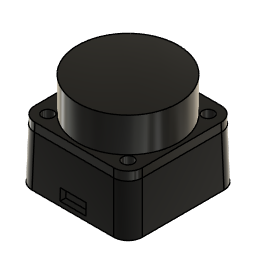
OKDO Lidar v2 (Autodesk Fusion 360 design; units mm, degrees)
Autodesk Fusion 360 part; units mm, degrees
note: some values were not read from the file. Set by a fixed rule: which face or edge a step refers to.
sketch "Sketch1" plane through (0, 0, 0) normal (0, 0, 1) x (1, 0, 0)
  line L0 (18.75, -18.75) -> (-18.75, -18.75)
  line L1 (-18.75, -18.75) -> (-18.75, 18.75)
  line L2 (-18.75, 18.75) -> (18.75, 18.75)
  line L3 (18.75, 18.75) -> (18.75, -18.75)
  line L4 (18.75, -18.75) -> (-18.75, 18.75) construction
  line L5 (-18.75, -18.75) -> (18.75, 18.75) construction
  dimension "d1" = 37.5
  dimension "d2" = 37.5
  constraint horizontal L0
  constraint perpendicular L0 L1
  constraint parallel L0 L2
  constraint parallel L1 L3
  constraint coincident L4 origin
  constraint coincident L5 origin
  measures "d1" distance of L1.end L2.end
  measures "d2" distance of L0.end L1.end
extrude "Extrude1" add sketch "Sketch1" against normal blind 20.5 makes body 1
sketch "Sketch2" plane through (0, 0, -20.5) normal (0, 0, -1) x (1, 0, 0)
  line L0 (-18.75, -18.75) -> (18.75, -18.75)
  line L1 (18.75, -18.75) -> (18.75, 18.75)
  line L2 (18.75, 18.75) -> (-18.75, 18.75)
  line L3 (-18.75, 18.75) -> (-18.75, -18.75)
  line L4 (19.25, 19.25) -> (-19.25, 19.25)
  line L5 (-19.25, 19.25) -> (-19.25, -19.25)
  line L6 (-19.25, -19.25) -> (19.25, -19.25)
  line L7 (19.25, -19.25) -> (19.25, 19.25)
  line L8 (19.25, 19.25) -> (-19.25, -19.25) construction
  line L9 (-19.25, 19.25) -> (19.25, -19.25) construction
  dimension "d5" = 38.5
  dimension "d6" = 38.5
  constraint horizontal L4
  constraint perpendicular L4 L5
  constraint parallel L4 L6
  constraint parallel L5 L7
  constraint coincident L8 origin
  constraint coincident L9 origin
  measures "d5" distance of L5.end L6.end
  measures "d6" distance of L4.end L5.end
sketch "Sketch3" plane through (0, -18.75, 0) normal (0, -1, 0) x (1, 0, 0)
  line L0 (18.75, 0) -> (-18.75, 0)
  line L1 (-18.75, 0) -> (-18.75, -20.5)
  line L2 (-18.75, -20.5) -> (18.75, -20.5)
  line L3 (18.75, -20.5) -> (18.75, 0)
  line L4 (-18.75, 0) -> (-19.25, -20.5)
  line L5 (-19.25, -20.5) -> (-18.75, -20.5)
  constraint coincident L0.end L1.start
  constraint coincident L1.end L2.start
extrude "Extrude2" add sketch "Sketch3" against normal blind 37.5 contours L1 L4 L5 bodies 1
pattern_circular "C-Pattern1" count 4 over 360 about axis through (0, 0, 1.75) along (0, 0, 1) of bodies 1 makes body 2 at (-6.25, -18.9167, -6.8333) makes body 3 at (18.9167, -6.25, -6.8333) makes body 4 at (6.25, 18.9167, -6.8333)
combine "Combine1" operation add target body 1 tool bodies 2 3 4
extrude "Extrude3" add 1 faces at (18.75, -18.9167, -13.6667) along direction (1, 0, 0) blind 0.9 on bodies 1 bodies 1
extrude "Extrude4" cut 1 faces at (19.2167, -18.75, -6.8333) along direction (0, -1, 0) blind 1.5 on bodies 1 bodies 1
extrude "Extrude5" add 1 faces at (18.75, 18.9167, -13.6667) along direction (1, 0, 0) blind 1 on bodies 1 bodies 1
extrude "Extrude6" add 2 faces at (-18.75, 18.9167, -13.6667) (-18.75, -18.9167, -13.6667) along direction (-1, 0, 0) blind 2.5 on bodies 1 bodies 1
extrude "Extrude7" cut 1 faces at (-19.75, -18.75, -6.8333) along direction (0, -1, 0) blind 11 on bodies 1 bodies 1
extrude "Extrude8" cut 1 faces at (-19.75, 18.75, -6.8333) along direction (0, 1, 0) blind 6 on bodies 1 bodies 1
extrude "Extrude9" cut 1 faces at (19.25, 18.75, -6.8333) along direction (0, 1, 0) blind 9 on bodies 1 bodies 1
sketch "Sketch4" plane through (0, 0, 0) normal (0, 0, 1) x (-1, 0, 0)
  line L0 (-18.75, -18.75) -> (18.75, -18.75)
  line L1 (18.75, -18.75) -> (18.75, 18.75)
  line L2 (18.75, 18.75) -> (-18.75, 18.75)
  line L3 (-18.75, 18.75) -> (-18.75, -18.75)
  circle A0 centre (0, 0) radius 17.5
  dimension "d25" = 35
  constraint coincident A0.centre origin
  measures "d25" diameter of A0
extrude "Extrude10" add sketch "Sketch4" along normal blind 12 contours A0 bodies 1
sketch "Sketch5" plane through (0, 0, 0) normal (0, 0, 1) x (-1, 0, 0)
  circle A0 centre (0, 0) radius 17.5
  line L0 (-18.75, -18.75) -> (18.75, -18.75)
  line L1 (18.75, -18.75) -> (18.75, 18.75)
  line L2 (18.75, 18.75) -> (-18.75, 18.75)
  line L3 (-18.75, 18.75) -> (-18.75, -18.75)
  line L4 (-14, -14) -> (14, -14)
  line L5 (14, -14) -> (14, 14)
  line L6 (14, 14) -> (-14, 14)
  line L7 (-14, 14) -> (-14, -14)
  line L8 (-14, -14) -> (14, 14) construction
  line L9 (14, -14) -> (-14, 14) construction
  circle A1 centre (14, -14) radius 2
  circle A2 centre (-14, -14) radius 2
  circle A3 centre (-14, 14) radius 2
  circle A4 centre (14, 14) radius 2
  dimension "d28" = 28
  dimension "d29" = 28
  dimension "d30" = 4
  dimension "d31" = 4
  dimension "d32" = 4
  dimension "d33" = 4
  constraint horizontal L4
  constraint perpendicular L4 L5
  constraint parallel L4 L6
  constraint parallel L5 L7
  constraint coincident L8 A0.centre
  constraint coincident L9 A0.centre
  constraint coincident A0.centre origin
  constraint coincident L4.end L5.start
  constraint coincident L4.start L7.end
  constraint coincident L6.end L7.start
  constraint coincident L5.end L6.start
  measures "d28" distance of L5.end L6.end
  measures "d29" distance of L4.end L5.end
  measures "d30" diameter of A1
  measures "d31" diameter of A2
  measures "d32" diameter of A3
  measures "d33" diameter of A4
extrude "Extrude11" cut sketch "Sketch5" against normal blind 20.5 contours L5 L6 A4 | L5 L6 A4 | L4 L5 A1 | L4 L5 A1 | L6 L7 A3 | L6 L7 A3 | L4 L7 A2 | L4 L7 A2 bodies 1
delete_face "DeleteFace1" 1 faces at (19.0833, 6.25, -20.5) on bodies 1
delete_face "DeleteFace2" 1 faces at (-6.25, -19.0833, -20.5) on bodies 1
delete_face "DeleteFace3" 1 faces at (-18.9166, -6.5833, -20.5) on bodies 1
delete_face "DeleteFace4" 1 faces at (-6.4167, 18.9178, -20.5) on bodies 1
ref_plane "WorkPlane1" through (0, 0, -3) normal (0, 0, 1) x (1, 0, 0)
split "Split1" by plane through (0, 0, -3) normal (0, 0, 1) bodies 1 makes body 5 at (-17.4782, 0.8723, 8)
fillet "Fillet1" radius 5 8 edges at (-19.0366, 19.0366, -11.75) (-19.0366, -19.0366, -11.75) (19.0366, 19.0366, -11.75) (19.0366, -19.0366, -11.75) (-18.7866, 18.7866, -1.5) (-18.7866, -18.7866, -1.5) (18.7866, 18.7866, -1.5) (18.7866, -18.7866, -1.5) on bodies 1 5
sketch "Sketch6" plane through (0, -18.7389, 0.457) normal (0, -0.999703, 0.024383) x (1, 0, 0)
  line L0 (14.2515, -20.9633) -> (13.8247, -3.4581)
  line L1 (13.8247, -3.4581) -> (-13.8247, -3.4581)
  line L2 (-13.8247, -3.4581) -> (-14.2515, -20.9633)
  line L3 (-14.2515, -20.9633) -> (14.2515, -20.9633)
  line L4 (0, -20.9633) -> (4.5, -20.9633)
  line L5 (4.5, -20.9633) -> (4.5, -19.4633)
  line L6 (4.5, -19.4633) -> (4.5, -15.4633)
  line L7 (4.5, -15.4633) -> (-4.5, -15.4633)
  line L8 (-4.5, -15.4633) -> (-4.5, -19.4633)
  line L9 (-4.5, -19.4633) -> (4.5, -19.4633)
  dimension "d39" = 4.5
  dimension "d40" = 1.5
  dimension "d41" = 4
  dimension "d42" = 9
  dimension "d43" = 4
  constraint midpoint L3 L4.start
  constraint parallel L3 L4
  constraint perpendicular L4 L5
  constraint parallel L5 L6
  constraint perpendicular L6 L7
  constraint perpendicular L7 L8
  measures "d39" distance of L4.start L4.end
  measures "d40" distance of L4.end L5.end
  measures "d41" distance of L5.end L6.end
  measures "d42" distance of L6.end L7.end
  measures "d43" distance of L7.end L8.end
extrude "Extrude12" cut sketch "Sketch6" against normal blind 2 contours L6 L7 L8 L9 bodies 1
sketch "Sketch7" plane through (0, 0, -20.5) normal (0, 0, -1) x (1, 0, 0)
  ellipse E0 centre (14.2485, 14.2485) end of major axis (17.7862, 17.7862) minor radius 5 (19.25, 14.2515) -> (14.2515, 19.25) ccw
  line L0 (14.2515, 19.25) -> (-14.2515, 19.25)
  ellipse E1 centre (-14.2485, 14.2485) end of major axis (-17.7862, 17.7862) minor radius 5 (-14.2515, 19.25) -> (-19.25, 14.2515) ccw
  line L1 (-19.25, 14.2515) -> (-19.25, -14.2515)
  ellipse E2 centre (-14.2485, -14.2485) end of major axis (-17.7862, -17.7862) minor radius 5 (-19.25, -14.2515) -> (-14.2515, -19.25) ccw
  line L2 (-14.2515, -19.25) -> (14.2515, -19.25)
  ellipse E3 centre (14.2485, -14.2485) end of major axis (17.7862, -17.7862) minor radius 5 (14.2515, -19.25) -> (19.25, -14.2515) ccw
  line L3 (19.25, -14.2515) -> (19.25, 14.2515)
  circle A0 centre (-14, 14) radius 2
  circle A1 centre (-14, -14) radius 2
  circle A2 centre (14, 14) radius 2
  circle A3 centre (14, -14) radius 2
  circle A4 centre (14, 14) radius 2.5
  circle A5 centre (-14, -14) radius 2.5
  dimension "d46" = 5
  dimension "d47" = 5
  constraint concentric A2 A4
  constraint concentric A1 A5
  measures "d46" diameter of A4
  measures "d47" diameter of A5
extrude "Extrude13" cut sketch "Sketch7" against normal blind 10 contours A4 | A5 bodies 1
sketch "Sketch8" plane through (0, 0, -20.5) normal (0, 0, -1) x (1, 0, 0)
  circle A0 centre (-14, -14) radius 2.5
  circle A1 centre (14, 14) radius 2.5
  ellipse E0 centre (14.2485, 14.2485) end of major axis (17.7862, 17.7862) minor radius 5 (19.25, 14.2515) -> (14.2515, 19.25) ccw
  line L0 (14.2515, 19.25) -> (-14.2515, 19.25)
  ellipse E1 centre (-14.2485, 14.2485) end of major axis (-17.7862, 17.7862) minor radius 5 (-14.2515, 19.25) -> (-19.25, 14.2515) ccw
  line L1 (-19.25, 14.2515) -> (-19.25, -14.2515)
  ellipse E2 centre (-14.2485, -14.2485) end of major axis (-17.7862, -17.7862) minor radius 5 (-19.25, -14.2515) -> (-14.2515, -19.25) ccw
  line L2 (-14.2515, -19.25) -> (14.2515, -19.25)
  ellipse E3 centre (14.2485, -14.2485) end of major axis (17.7862, -17.7862) minor radius 5 (14.2515, -19.25) -> (19.25, -14.2515) ccw
  line L3 (19.25, -14.2515) -> (19.25, 14.2515)
  circle A2 centre (-14, 14) radius 2
  circle A3 centre (14, -14) radius 2
  circle A4 centre (-14, 14) radius 2
  circle A5 centre (14, -14) radius 2
  constraint concentric A2 A4
  constraint concentric A3 A5
extrude "Extrude14" add sketch "Sketch8" against normal blind 13 contours A2 A4 | A3 A5 bodies 1
